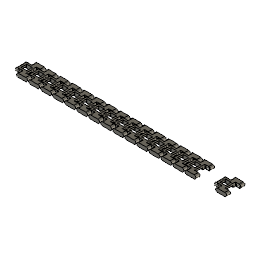
hinge_s (Autodesk Fusion 360 design; units mm, degrees)
Autodesk Fusion 360 part; units mm, degrees
note: some values were not read from the file. Chosen so that the rebuilt part matches the saved one: that a step has no effect; which sketch regions a step uses.
sketch "スケッチ1" plane through (0, 0, 0) normal (0, 0, 1) x (1, 0, 0)
  line L0 (0, 0) -> (0, 2.5)
  line L1 (0, 2.5) -> (3, 2.5)
  line L2 (3, 2.5) -> (3, 5)
  line L3 (3, 5) -> (9, 5)
  line L4 (9, 5) -> (9, 2.8)
  line L5 (9, 2.8) -> (6, 2.8)
  line L6 (6, 2.8) -> (6, -2.8)
  line L7 (6, -2.8) -> (9, -2.8)
  line L8 (9, -2.8) -> (9, -5)
  line L9 (9, -5) -> (3, -5)
  line L10 (3, -5) -> (3, -2.5)
  line L11 (3, -2.5) -> (0, -2.5)
  line L12 (0, -2.5) -> (0, 0)
  line L13 (3, 1.5013) -> (5, 1.5013)
  line L14 (5, 1.5013) -> (5, -1.5)
  line L15 (5, -1.5) -> (2, -1.5)
  line L16 (2, -1.5) -> (2, 1.5013)
  line L17 (2, 1.5013) -> (3, 1.5013)
  constraint coincident L0.start L12.end
  constraint perpendicular L0 L1
  constraint perpendicular L1 L2
  constraint perpendicular L2 L3
  constraint perpendicular L3 L4
  constraint perpendicular L4 L5
  constraint perpendicular L5 L6
  constraint perpendicular L4 L7
  constraint perpendicular L5 L8
  constraint perpendicular L8 L9
  constraint perpendicular L5 L10
  constraint perpendicular L8 L11
  constraint perpendicular L11 L12
  constraint perpendicular L13 L14
  constraint perpendicular L14 L15
  constraint perpendicular L13 L16
  constraint perpendicular L16 L17
combine "結合1" [no effect]
combine "結合2" [no effect]
extrude "押し出し12" [no effect]
extrude "押し出し13" [no effect]
extrude "押し出し14" cut sketch "スケッチ1" along normal blind 2 contours L13 L14 L15 L16 L17
extrude "押し出し15" [no effect]
extrude "押し出し16" [no effect]
extrude "押し出し21" [no effect]
extrude "押し出し22" [no effect]
extrude "押し出し23" [no effect]
extrude "押し出し24" [no effect]
extrude "押し出し25" [no effect]
extrude "押し出し26" [no effect]
combine "結合4" [no effect]
extrude "押し出し27" add sketch "スケッチ1" along normal blind 2 separate body makes body 1
sketch "スケッチ14" plane through (0, 2.8, 0) normal (0, -1, 0) x (1, 0, 0)
  line L0 (6, 0) -> (9, 0)
  line L1 (9, 0) -> (9, 2)
  line L2 (9, 2) -> (6, 2)
  line L3 (6, 2) -> (6, 0)
  circle A0 centre (7.5, 1) radius 1
  dimension "d66" = 2
  measures "d66" diameter of A0
sketch "スケッチ15" plane through (0, -2.8, 0) normal (0, 1, 0) x (-1, 0, 0)
  line L0 (-9, 0) -> (-6, 0)
  line L1 (-6, 0) -> (-6, 2)
  line L2 (-6, 2) -> (-9, 2)
  line L3 (-9, 2) -> (-9, 0)
  circle A0 centre (-7.5, 1) radius 1
  dimension "d67" = 2
  measures "d67" diameter of A0
sketch "スケッチ16" plane through (0, 2.5, 0) normal (0, 1, 0) x (-1, 0, 0)
  line L0 (-3, 0) -> (0, 0)
  line L1 (0, 0) -> (0, 2)
  line L2 (0, 2) -> (-3, 2)
  line L3 (-3, 2) -> (-3, 0)
  circle A0 centre (-1, 1) radius 1
  dimension "d68" = 2
  measures "d68" diameter of A0
sketch "スケッチ17" plane through (0, -2.5, 0) normal (0, -1, 0) x (1, 0, 0)
  line L0 (0, 0) -> (3, 0)
  line L1 (3, 0) -> (3, 2)
  line L2 (3, 2) -> (0, 2)
  line L3 (0, 2) -> (0, 0)
  circle A0 centre (1.0104, 1) radius 1
  dimension "d69" = 2
  measures "d69" diameter of A0
extrude "押し出し28" cut sketch "スケッチ14" against normal blind 3 draft -30 contours A0 bodies 1
extrude "押し出し29" cut sketch "スケッチ15" against normal blind 3 draft -30 contours A0 bodies 1
extrude "押し出し30" add sketch "スケッチ16" along normal blind 3 draft -35 contours A0 bodies 1
extrude "押し出し31" add sketch "スケッチ17" along normal blind 3 draft -35 contours A0 bodies 1
sketch "スケッチ18" plane through (0, 0, 0) normal (0, 0, 1) x (1, 0, 0)
  line L0 (0, 1.5) -> (6, 1.5)
  line L1 (6, 1.5) -> (6, -1.5)
  line L2 (6, -1.5) -> (0, -1.5)
  line L3 (0, -1.5) -> (0, 1.5)
  constraint horizontal L0
  constraint vertical L1
  constraint horizontal L2
  constraint vertical L3
extrude "押し出し32" cut sketch "スケッチ18" along normal blind 1 bodies 1
fillet "フィレット4" radius 1 11 edges at (0, 0, 2) (3, -3.75, 2) (9, -3.9, 2) (9, 3.9, 2) (3, 3.75, 2) (9, 3.9, 0) (9, -3.9, 0) (3, 3.75, 0) (3, -3.75, 0) (0, -2, 0) (0, 2, 0) on bodies 1
copy_body "ボディのコピーと貼り付け35" bodies 1 makes body 2
move_body "移動37" bodies 2 to x (1, 0, 0) y (0, 1, 0) z (0, 0, 1) at (6.5, 0, 0)
copy_body "ボディのコピーと貼り付け36" bodies 2 1 makes body 3 makes body 4
move_body "移動38" bodies 3 4 to x (1, 0, 0) y (0, 1, 0) z (0, 0, 1) at (13, 0, 0)
copy_body "ボディのコピーと貼り付け37" bodies 3 1 2 4 makes body 5 makes body 6 makes body 7 makes body 8
move_body "移動39" bodies 5 6 7 8 to x (1, 0, 0) y (0, 1, 0) z (0, 0, 1) at (26, 0, 0)
copy_body "ボディのコピーと貼り付け38" bodies 8 1 4 2 5 3 7 6 makes body 9 makes body 10 makes body 11 makes body 12 makes body 13 makes body 14 makes body 15 makes body 16
move_body "移動40" bodies 9 10 11 12 13 14 15 16 to x (1, 0, 0) y (0, 1, 0) z (0, 0, 1) at (52, 0, 0)
move_body "移動41" bodies 13 to x (1, 0, 0) y (0, 1, 0) z (0, 0, 1) at (10, 0, 0)
